spool_cradle_bracket (Autodesk Fusion 360 design; units mm, degrees)
part number: 2026-09-02-15-56-20-841
Autodesk Fusion 360 part; units mm, degrees
sketch "Arm triangle" plane through (0, 0, 0) normal (0, 1, 0) x (1, 0, 0)
  line L0 (0, 0) -> (0, -90)
  line L1 (0, -90) -> (150, -90)
  line L2 (150, -90) -> (0, 0)
extrude "Arm triangle (1)" add sketch "Arm triangle" along normal mid plane 24
sketch "Hook plate" plane through (0, 0, 0) normal (0, 1, 0) x (1, 0, 0)
  line L0 (0, 0) -> (6, 0)
  line L1 (6, 0) -> (6, -90)
  line L2 (6, -90) -> (0, -90)
  line L3 (0, -90) -> (0, 0)
extrude "Hook plate (1)" add sketch "Hook plate" along normal mid plane 24
sketch "Lightening cutout" plane through (0, 0, 0) normal (0, 1, 0) x (1, 0, 0)
  line L0 (14, -24.7267) -> (14, -76)
  line L1 (14, -76) -> (37.3, -76)
  line L2 (37.3, -76) -> (37.3, -38.7067)
  line L3 (37.3, -38.7067) -> (14, -24.7267)
extrude "Lightening cutout (1)" cut sketch "Lightening cutout" along normal mid plane 34
sketch "Saddle boss x=70" plane through (0, 0, 0) normal (0, 1, 0) x (1, 0, 0)
  circle A0 centre (70, -90) radius 22.7
extrude "Saddle boss x=70 (1)" add sketch "Saddle boss x=70" along normal mid plane 24
sketch "Saddle boss x=150" plane through (0, 0, 0) normal (0, 1, 0) x (1, 0, 0)
  circle A0 centre (150, -90) radius 22.7
extrude "Saddle boss x=150 (1)" add sketch "Saddle boss x=150" along normal mid plane 24
sketch "Rod pocket x=70" plane through (0, 0, 0) normal (0, 1, 0) x (1, 0, 0)
  circle A0 centre (70, -90) radius 17.1
extrude "Rod pocket x=70 (1)" cut sketch "Rod pocket x=70" along normal mid plane 34
sketch "Drop-in opening x=70" plane through (0, 0, 0) normal (0, 1, 0) x (1, 0, 0)
  line L0 (52.9, -90) -> (87.1, -90)
  line L1 (87.1, -90) -> (87.1, -117.7)
  line L2 (87.1, -117.7) -> (52.9, -117.7)
  line L3 (52.9, -117.7) -> (52.9, -90)
extrude "Drop-in opening x=70 (1)" cut sketch "Drop-in opening x=70" along normal mid plane 34
sketch "Rod pocket x=150" plane through (0, 0, 0) normal (0, 1, 0) x (1, 0, 0)
  circle A0 centre (150, -90) radius 17.1
extrude "Rod pocket x=150 (1)" cut sketch "Rod pocket x=150" along normal mid plane 34
sketch "Drop-in opening x=150" plane through (0, 0, 0) normal (0, 1, 0) x (1, 0, 0)
  line L0 (132.9, -90) -> (167.1, -90)
  line L1 (167.1, -90) -> (167.1, -117.7)
  line L2 (167.1, -117.7) -> (132.9, -117.7)
  line L3 (132.9, -117.7) -> (132.9, -90)
extrude "Drop-in opening x=150 (1)" cut sketch "Drop-in opening x=150" along normal mid plane 34
sketch "Hook profile" plane through (0, 0, 0) normal (0, 1, 0) x (1, 0, 0)
  line L0 (0, -88) -> (-8.3, -88)
  line L1 (-8.3, -88) -> (-8.3, -71)
  line L2 (-8.3, -71) -> (-5.3, -71)
  line L3 (-5.3, -71) -> (-3.8, -72.5)
  line L4 (-3.8, -72.5) -> (-3.8, -83)
  line L5 (-3.8, -83) -> (0, -83)
  line L6 (0, -83) -> (0, -88)
  dimension "d82" = 88
  dimension "d83" = 8.3
  dimension "d84" = 3.8
  dimension "d85" = 5
  dimension "d86" = 10.5
  dimension "d87" = 1.5
  dimension "d88" = 1.5
  constraint horizontal L0
  constraint horizontal L2
  constraint horizontal L5
  constraint vertical L1
  constraint vertical L4
  constraint vertical L6
  constraint coincident origin L6
  measures "d82" vertical distance of origin L0.start
  measures "d83" horizontal distance of L0.start L0.end
  measures "d84" horizontal distance of L4.end L5.end
  measures "d85" vertical distance of L0.start L5.end
  measures "d86" vertical distance of L3.end L4.end
  measures "d87" horizontal distance of L2.end L3.end
  measures "d88" vertical distance of L2.end L3.end
extrude "Hook profile (1)" add sketch "Hook profile" along normal mid plane 2.4
pattern_linear "Hook rows" count 4 spacing 25.4 along (0, 0, -1) count 3 spacing 0 along (0, 0, 1) of "Hook profile (1)"
equation "bracketWidth = 24.0 mm" comment "drives the model; safe to edit live in Fusion"
equation "couponWidth = 8.0 mm" comment "drives the model; safe to edit live in Fusion"
equation "hookTabWidth = 2.4 mm" comment "drives the model; safe to edit live in Fusion"
equation "slotHeight = 19.05 mm" comment "reference only â edit scripts/build_rod_bracket.py and rebuild"
equation "slotPitchVertical = 25.4 mm" comment "drives the model; safe to edit live in Fusion"
equation "slotWidth = 3.2 mm" comment "reference only â edit scripts/build_rod_bracket.py and rebuild"
equation "faceMetalThickness = 2.0 mm" comment "drives the model; safe to edit live in Fusion"
equation "hookThroat = faceMetalThickness + 1.8 mm" comment "drives the model; safe to edit live in Fusion"
equation "hookNeckHeight = 5.0 mm" comment "drives the model; safe to edit live in Fusion"
equation "hookLipThickness = 4.5 mm" comment "drives the model; safe to edit live in Fusion"
equation "hookLipDrop = 12.0 mm" comment "drives the model; safe to edit live in Fusion"
equation "plateThickness = 6.0 mm" comment "reference only â edit scripts/build_rod_bracket.py and rebuild"
equation "plateHeight = 90.0 mm" comment "reference only â edit scripts/build_rod_bracket.py and rebuild"
equation "gaugePlateThickness = 5.0 mm" comment "reference only â edit scripts/build_rod_bracket.py and rebuild"
equation "rodOuterDiameter = 33.4 mm" comment "reference only â edit scripts/build_rod_bracket.py and rebuild"
equation "saddleClearance = 0.8 mm" comment "reference only â edit scripts/build_rod_bracket.py and rebuild"
equation "saddleWall = 6.0 mm" comment "reference only â edit scripts/build_rod_bracket.py and rebuild"
equation "rearRodStandoff = 70.0 mm" comment "reference only â edit scripts/build_rod_bracket.py and rebuild"
equation "rodSpacing = 80.0 mm" comment "reference only â edit scripts/build_rod_bracket.py and rebuild"
equation "memberWidth = 14.0 mm" comment "reference only â edit scripts/build_rod_bracket.py and rebuild"
equation "hookLipChamfer = 1.5 mm" comment "drives the model; safe to edit live in Fusion"
equation "topHookNeckTop = 88.0 mm" comment "drives the model; safe to edit live in Fusion"
equation "hookRows = 4" comment "drives the model; safe to edit live in Fusion"
equation "d64 = bracketWidth"
equation "d66 = bracketWidth"
equation "d68 = bracketWidth + 10 mm"
equation "d70 = bracketWidth"
equation "d72 = bracketWidth"
equation "d74 = bracketWidth + 10 mm"
equation "d76 = bracketWidth + 10 mm"
equation "d78 = bracketWidth + 10 mm"
equation "d80 = bracketWidth + 10 mm"
equation "d82 = topHookNeckTop"
equation "d83 = hookThroat + hookLipThickness"
equation "d84 = hookThroat"
equation "d85 = hookNeckHeight"
equation "d86 = hookLipDrop - hookLipChamfer"
equation "d87 = hookLipChamfer"
equation "d88 = hookLipChamfer"
equation "d89 = hookTabWidth"
equation "d91 = hookRows"
equation "d93 = -slotPitchVertical"
named bodies: "spool_cradle_bracket"
